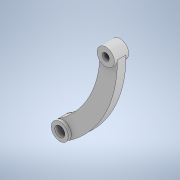
# Autodesk Inventor part: tolo
Saved by Autodesk Inventor 2020 (Build 240168000, 168)
## iProperties
Created: 2019-08-11
Part Number: tolo
Material: Generic
Document SubType Name: Modeling
Designer: Horváth Patrik
Density: 1 g/cm^3
Appearance: Default
Author: Horváth Patrik
Autodesk Inventor part; units mm, degrees
ref_plane "YZ Plane" through (0, 0, 0) normal (1, 0, 0) x (0, 1, 0)
ref_plane "XZ Plane" through (0, 0, 0) normal (0, 1, 0) x (-1, 0, 0)
ref_plane "XY Plane" through (0, 0, 0) normal (0, 0, 1) x (1, 0, 0)
sketch "Sketch2" plane through (0, 0, 0) normal (0, 0, 1) x (1, 0, 0)
  circle A0 centre (21.7341, 34.515) radius 1.25
  arc A1 (5.7341, 4.015) -> (21.7341, 34.515) centre (-14.2615, 33.9512) ccw construction
  arc A2 (7.4004, 1.5204) -> (24.7337, 34.562) centre (-14.2615, 33.9512) ccw
  arc A3 (4.0678, 6.5097) -> (18.7344, 34.4681) centre (-14.2615, 33.9512) ccw
  arc A4 (4.0678, 6.5097) -> (7.4004, 1.5204) centre (5.7341, 4.015) ccw
  arc A5 (24.7337, 34.562) -> (18.7344, 34.4681) centre (21.7341, 34.515) ccw
  circle A6 centre (5.7341, 4.015) radius 1.75
  dimension "d18" = 6
  dimension "d21" = 33
  dimension "d22" = 30.5
  dimension "d23" = 16
  dimension "d24" = 2.5
  dimension "d26" = 3.5
  constraints: 10 point on circle, 7 centre point, 4 tangent, 2 coincident
  measures "d18" radial gap between concentric circles of A2 A3
  measures "d21" radius of A3
  measures "d22" vertical distance of A0.centre point (5.734, 4.015)
  measures "d23" horizontal distance of A0.centre point (5.734, 4.015)
  measures "d24" diameter of A0
  measures "d26" diameter of A6
extrude "Extrusion1" add sketch "Sketch2" along normal mid plane 3
sketch "Sketch3" plane through (0, 0, 1.5) normal (0, 0, 1) x (1, 0, 0)
  arc A0 (4.0678, 6.5097) -> (7.4004, 1.5204) centre (5.7341, 4.015) ccw projected
  arc A1 (24.7337, 34.562) -> (18.7344, 34.4681) centre (21.7341, 34.515) ccw projected
  circle A2 centre (5.7341, 4.015) radius 1.75 projected
  circle A3 centre (21.7341, 34.515) radius 1.25 projected
  circle A4 centre (5.7341, 4.015) radius 3
  circle A5 centre (21.7341, 34.515) radius 3
  point P0 (0, 0)
  point P1 (18.7344, 34.4681)
  point P2 (24.7337, 34.562)
  point P3 (7.4004, 1.5204)
  point P4 (4.0678, 6.5097)
  constraints: 2 centre point, 2 coincident, 2 concentric
extrude "Extrusion2" add sketch "Sketch3" along normal blind 1
mirror "Mirror1" about plane through (0, 0, 0) normal (0, 0, 1) of "Extrusion2"
body "Solid1"
